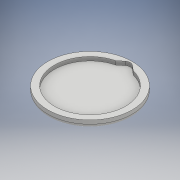
# Autodesk Inventor part: CalorimeterCap
Saved by Autodesk Inventor 2018 (Build 220112000, 112)
## iProperties
Created: 2020-04-09
Part Number: CalorimeterCap
Material: Generic
Document SubType Name: Modeling
Designer: Ivan
Density: 1 g/cm^3
Appearance: Default
Author: Ivan
Autodesk Inventor part; units mm, degrees
ref_plane "YZ Plane" through (0, 0, 0) normal (1, 0, 0) x (0, 1, 0)
ref_plane "XZ Plane" through (0, 0, 0) normal (0, 1, 0) x (-1, 0, 0)
ref_plane "XY Plane" through (0, 0, 0) normal (0, 0, 1) x (1, 0, 0)
sketch "Sketch1" plane through (0, 0, 0) normal (0, 0, 1) x (1, 0, 0)
  circle A0 centre (0, 0) radius 56
  dimension "d0" = 112
  constraints: 1 centre point, 1 coincident
  measures "d0" diameter of A0
extrude "Extrusion1" add sketch "Sketch1" along normal blind 10
sketch "Sketch2" plane through (0, 0, 10) normal (0, 0, 1) x (1, 0, 0)
  circle A0 centre (0, 0) radius 47.5
  dimension "d4" = 95
  constraints: 1 centre point, 1 coincident
  measures "d4" diameter of A0
extrude "Extrusion2" cut sketch "Sketch2" against normal blind 5
sketch "Sketch3" plane through (0, 0, 10) normal (0, 0, 1) x (1, 0, 0)
  circle A0 centre (0, 0) radius 56 projected
  circle A1 centre (0, 0) radius 56 construction
  line L0 (0, 56) -> (0, 48.5) construction
  circle A2 centre (0, 0) radius 47.5 construction
  arc A3 (11.5918, 46.0639) -> (-11.5918, 46.0639) centre (0, 0) ccw
  arc A4 (4.8209, 51.7453) -> (-4.8209, 51.7453) centre (0, 46) ccw
  line L1 (-4.8209, 51.7453) -> (-11.5918, 46.0639)
  line L2 (4.8209, 51.7453) -> (11.5918, 46.0639)
  point P0 (-16.2948, 44.6176)
  point P1 (-7.3339, 46.9304)
  point P2 (7.3339, 46.9304)
  point P3 (16.2948, 44.6176)
  dimension "d12" = 15
  dimension "d13" = 10
  dimension "d15" = 50
  constraints: 6 end point, 6 point on circle, 3 symmetric about line, 3 vertical alignment, 2 centre point, 1 coincident, 1 tangent, 1 vertical, 4 other
  measures "d12" diameter of A4
  measures "d13" distance of L0.start A4.centre
  measures "d15" angle of L0 L1
extrude "Extrusion4" cut sketch "Sketch3" against normal up to surface (5 mm away) contours A3 L1 A4 L2
fillet "Fillet1" radius 5 1 edges at (-56, 0, 0)
body "Solid1"
